Autodesk Inventor part; units mm, degrees
(part 2 of 3)
  spline S229 degree 2 poles (-22.9863, 76.6126) (-22.9863, 77.0351) (-22.389, 77.6357) (-21.9632, 77.6357) knots 0 0 0 1 2 2 2
  line L306 (-21.9632, 77.6357) -> (-21.1876, 77.6357)
  spline S230 degree 2 poles (-21.1876, 77.6357) (-20.9335, 77.6357) (-20.9335, 77.3882) knots 0 0 0 1 1 1
  spline S231 degree 2 poles (-20.9335, 77.3882) (-20.9335, 77.1374) (-21.1876, 77.1374) knots 0 0 0 1 1 1
  line L307 (-21.1876, 77.1374) -> (-21.9632, 77.1374)
  spline S232 degree 2 poles (-21.9632, 77.1374) (-22.1777, 77.1374) (-22.4847, 76.8304) (-22.4847, 76.6126) knots 0 0 0 1 2 2 2
  line L308 (-22.4847, 76.6126) -> (-22.4847, 74.672)
  spline S233 degree 2 poles (-22.4847, 74.672) (-22.4847, 74.4542) (-22.1777, 74.1473) (-21.9632, 74.1473) knots 0 0 0 1 2 2 2
  line L309 (-21.9632, 74.1473) -> (-21.1876, 74.1473)
  spline S234 degree 2 poles (-21.1876, 74.1473) (-20.9335, 74.1473) (-20.9335, 73.8997) knots 0 0 0 1 1 1
  spline S235 degree 2 poles (-20.9335, 73.8997) (-20.9335, 73.6489) (-21.1876, 73.6489) knots 0 0 0 1 1 1
  spline S236 degree 2 poles (-17.7355, 74.8667) (-17.7355, 74.3651) (-18.4517, 73.6489) (-18.9566, 73.6489) knots 0 0 0 1 2 2 2
  line L310 (-18.9566, 73.6489) -> (-20.1183, 73.6489)
  spline S237 degree 2 poles (-20.1183, 73.6489) (-20.2306, 73.6489) (-20.3692, 73.7875) (-20.3692, 73.8997) knots 0 0 0 1 2 2 2
  line L311 (-20.3692, 73.8997) -> (-20.3692, 77.3849)
  spline S238 degree 2 poles (-20.3692, 77.3849) (-20.3692, 77.4872) (-20.2207, 77.6357) (-20.1183, 77.6357) knots 0 0 0 1 2 2 2
  line L312 (-20.1183, 77.6357) -> (-18.9566, 77.6357)
  spline S239 degree 2 poles (-18.9566, 77.6357) (-18.5342, 77.6357) (-17.9302, 77.0318) (-17.9302, 76.6093) knots 0 0 0 1 2 2 2
  spline S240 degree 2 poles (-17.9302, 76.6093) (-17.9302, 76.1242) (-18.29, 75.8601) knots 0 0 0 1 1 1
  spline S241 degree 2 poles (-18.29, 75.8601) (-17.7355, 75.5433) (-17.7355, 74.8667) knots 0 0 0 1 1 1
  spline S242 degree 2 poles (-18.2372, 74.8667) (-18.2372, 75.1638) (-18.6596, 75.5862) (-18.9566, 75.5862) knots 0 0 0 1 2 2 2
  line L313 (-18.9566, 75.5862) -> (-19.8675, 75.5862)
  line L314 (-19.8675, 75.5862) -> (-19.8675, 74.1473)
  line L315 (-19.8675, 74.1473) -> (-18.9566, 74.1473)
  spline S243 degree 2 poles (-18.9566, 74.1473) (-18.6596, 74.1473) (-18.2372, 74.5697) (-18.2372, 74.8667) knots 0 0 0 1 2 2 2
  spline S244 degree 2 poles (-18.4319, 76.6126) (-18.4319, 76.8271) (-18.7421, 77.1374) (-18.9566, 77.1374) knots 0 0 0 1 2 2 2
  line L316 (-18.9566, 77.1374) -> (-19.8675, 77.1374)
  line L317 (-19.8675, 77.1374) -> (-19.8675, 76.0846)
  line L318 (-19.8675, 76.0846) -> (-18.9566, 76.0846)
  spline S245 degree 2 poles (-18.9566, 76.0846) (-18.7421, 76.0846) (-18.4319, 76.3948) (-18.4319, 76.6126) knots 0 0 0 1 2 2 2
  spline S246 degree 2 poles (-14.7289, 73.8997) (-14.7289, 73.6489) (-14.9797, 73.6489) knots 0 0 0 1 1 1
  spline S247 degree 2 poles (-14.9797, 73.6489) (-15.2306, 73.6489) (-15.2306, 73.8997) knots 0 0 0 1 1 1
  line L319 (-15.2306, 73.8997) -> (-15.2306, 75.2001)
  line L320 (-15.2306, 75.2001) -> (-15.8081, 75.2001)
  line L321 (-15.8081, 75.2001) -> (-16.7091, 73.7644)
  spline S248 degree 2 poles (-16.7091, 73.7644) (-16.7817, 73.6456) (-16.917, 73.6456) knots 0 0 0 1 1 1
  spline S249 degree 2 poles (-16.917, 73.6456) (-17.016, 73.6456) (-17.1744, 73.7941) (-17.1744, 73.8964) knots 0 0 0 1 2 2 2
  spline S250 degree 2 poles (-17.1744, 73.8964) (-17.1744, 73.9624) (-17.1348, 74.0285) knots 0 0 0 1 1 1
  line L322 (-17.1348, 74.0285) -> (-16.3428, 75.2463)
  spline S251 degree 2 poles (-16.3428, 75.2463) (-16.6794, 75.3123) (-17.1711, 75.9261) (-17.1711, 76.3222) knots 0 0 0 1 2 2 2
  line L323 (-17.1711, 76.3222) -> (-17.1711, 76.5136)
  spline S252 degree 2 poles (-17.1711, 76.5136) (-17.1711, 76.979) (-16.5144, 77.6357) (-16.049, 77.6357) knots 0 0 0 1 2 2 2
  line L324 (-16.049, 77.6357) -> (-14.983, 77.6357)
  spline S253 degree 2 poles (-14.983, 77.6357) (-14.8807, 77.6357) (-14.7289, 77.4839) (-14.7289, 77.3849) knots 0 0 0 1 2 2 2
  line L325 (-14.7289, 77.3849) -> (-14.7289, 73.8997)
  line L326 (-15.2306, 75.6984) -> (-15.2306, 77.1374)
  line L327 (-15.2306, 77.1374) -> (-16.049, 77.1374)
  spline S254 degree 2 poles (-16.049, 77.1374) (-16.3032, 77.1374) (-16.6695, 76.771) (-16.6695, 76.5136) knots 0 0 0 1 2 2 2
  line L328 (-16.6695, 76.5136) -> (-16.6695, 76.3222)
  spline S255 degree 2 poles (-16.6695, 76.3222) (-16.6695, 76.0648) (-16.3032, 75.6984) (-16.049, 75.6984) knots 0 0 0 1 2 2 2
  line L329 (-16.049, 75.6984) -> (-15.2306, 75.6984)
  spline S256 degree 2 poles (-12.016, 74.6753) (-12.016, 74.2496) (-12.6134, 73.6489) (-13.0424, 73.6489) knots 0 0 0 1 2 2 2
  line L330 (-13.0424, 73.6489) -> (-13.1381, 73.6489)
  spline S257 degree 2 poles (-13.1381, 73.6489) (-13.7355, 73.6489) (-14.0325, 74.1605) knots 0 0 0 1 1 1
  spline S258 degree 2 poles (-14.0325, 74.1605) (-14.0721, 74.2265) (-14.0721, 74.2892) knots 0 0 0 1 1 1
  spline S259 degree 2 poles (-14.0721, 74.2892) (-14.0721, 74.3915) (-13.9104, 74.54) (-13.8114, 74.54) knots 0 0 0 1 2 2 2
  spline S260 degree 2 poles (-13.8114, 74.54) (-13.6761, 74.54) (-13.6299, 74.4377) knots 0 0 0 1 1 1
  spline S261 degree 2 poles (-13.6299, 74.4377) (-13.4451, 74.1473) (-13.1381, 74.1473) knots 0 0 0 1 1 1
  line L331 (-13.1381, 74.1473) -> (-13.0424, 74.1473)
  spline S262 degree 2 poles (-13.0424, 74.1473) (-12.8246, 74.1473) (-12.5177, 74.4575) (-12.5177, 74.672) knots 0 0 0 1 2 2 2
  line L332 (-12.5177, 74.672) -> (-12.5177, 75.0615)
  spline S263 degree 2 poles (-12.5177, 75.0615) (-12.5177, 75.276) (-12.8279, 75.5862) (-13.0424, 75.5862) knots 0 0 0 1 2 2 2
  line L333 (-13.0424, 75.5862) -> (-13.4286, 75.5862)
  spline S264 degree 2 poles (-13.4286, 75.5862) (-13.6794, 75.5862) (-13.6794, 75.837) knots 0 0 0 1 1 1
  spline S265 degree 2 poles (-13.6794, 75.837) (-13.6794, 76.0846) (-13.4286, 76.0846) knots 0 0 0 1 1 1
  line L334 (-13.4286, 76.0846) -> (-12.8807, 76.0846)
  spline S266 degree 2 poles (-12.8807, 76.0846) (-12.7223, 76.1242) (-12.5177, 76.3915) (-12.5177, 76.5598) knots 0 0 0 1 2 2 2
  spline S267 degree 2 poles (-12.5177, 76.5598) (-12.5177, 76.8007) (-12.8576, 77.1374) (-13.0985, 77.1374) knots 0 0 0 1 2 2 2
  spline S268 degree 2 poles (-13.0985, 77.1374) (-13.3032, 77.1374) (-13.4649, 76.9988) knots 0 0 0 1 1 1
  spline S269 degree 2 poles (-13.4649, 76.9988) (-13.5408, 76.9393) (-13.6233, 76.9393) knots 0 0 0 1 1 1
  spline S270 degree 2 poles (-13.6233, 76.9393) (-13.7256, 76.9393) (-13.8774, 77.0978) (-13.8774, 77.1968) knots 0 0 0 1 2 2 2
  spline S271 degree 2 poles (-13.8774, 77.1968) (-13.8774, 77.3024) (-13.6893, 77.3948) knots 0 0 0 1 1 1
  spline S272 degree 2 poles (-13.6893, 77.3948) (-13.4814, 77.6357) (-13.0985, 77.6357) knots 0 0 0 1 1 1
  spline S273 degree 2 poles (-13.0985, 77.6357) (-12.6464, 77.6357) (-12.016, 77.0087) (-12.016, 76.5598) knots 0 0 0 1 2 2 2
  spline S274 degree 2 poles (-12.016, 76.5598) (-12.016, 76.0681) (-12.3791, 75.8172) knots 0 0 0 1 1 1
  spline S275 degree 2 poles (-12.3791, 75.8172) (-12.016, 75.5499) (-12.016, 75.0615) knots 0 0 0 1 1 1
  line L335 (-12.016, 75.0615) -> (-12.016, 74.6753)
  spline S276 degree 2 poles (-8.9104, 74.672) (-8.9104, 74.2463) (-9.5111, 73.6489) (-9.9401, 73.6489) knots 0 0 0 1 2 2 2
  line L336 (-9.9401, 73.6489) -> (-11.1018, 73.6489)
  spline S277 degree 2 poles (-11.1018, 73.6489) (-11.2041, 73.6489) (-11.3527, 73.7974) (-11.3527, 73.8997) knots 0 0 0 1 2 2 2
  line L337 (-11.3527, 73.8997) -> (-11.3527, 77.3849)
  spline S278 degree 2 poles (-11.3527, 77.3849) (-11.3527, 77.6357) (-11.1018, 77.6357) knots 0 0 0 1 1 1
  spline S279 degree 2 poles (-11.1018, 77.6357) (-10.851, 77.6357) (-10.851, 77.3849) knots 0 0 0 1 1 1
  line L338 (-10.851, 77.3849) -> (-10.851, 76.0846)
  line L339 (-10.851, 76.0846) -> (-9.9401, 76.0846)
  spline S280 degree 2 poles (-9.9401, 76.0846) (-9.5111, 76.0846) (-8.9104, 75.4839) (-8.9104, 75.0615) knots 0 0 0 1 2 2 2
  line L340 (-8.9104, 75.0615) -> (-8.9104, 74.672)
  line L341 (-9.4121, 74.672) -> (-9.4121, 75.0615)
  spline S281 degree 2 poles (-9.4121, 75.0615) (-9.4121, 75.276) (-9.7223, 75.5862) (-9.9401, 75.5862) knots 0 0 0 1 2 2 2
  line L342 (-9.9401, 75.5862) -> (-10.851, 75.5862)
  line L343 (-10.851, 75.5862) -> (-10.851, 74.1473)
  line L344 (-10.851, 74.1473) -> (-9.9401, 74.1473)
  spline S282 degree 2 poles (-9.9401, 74.1473) (-9.7223, 74.1473) (-9.4121, 74.4575) (-9.4121, 74.672) knots 0 0 0 1 2 2 2
  line L345 (-22.255, 49.6974) -> (-23.8504, 49.6974)
  spline S283 degree 2 poles (-23.8504, 49.6974) (-24.0502, 49.6974) (-24.0502, 49.8972) knots 0 0 0 1 1 1
  line L346 (-24.0502, 49.8972) -> (-24.0502, 53.4842)
  spline S284 degree 2 poles (-24.0502, 53.4842) (-24.0502, 53.6841) (-23.8504, 53.6841) knots 0 0 0 1 1 1
  spline S285 degree 2 poles (-23.8504, 53.6841) (-23.6506, 53.6841) (-23.6506, 53.4842) knots 0 0 0 1 1 1
  line L347 (-23.6506, 53.4842) -> (-23.6506, 50.0971)
  line L348 (-23.6506, 50.0971) -> (-22.255, 50.0971)
  spline S286 degree 2 poles (-22.255, 50.0971) (-22.0552, 50.0971) (-22.0552, 49.8972) knots 0 0 0 1 1 1
  spline S287 degree 2 poles (-22.0552, 49.8972) (-22.0552, 49.6974) (-22.255, 49.6974) knots 0 0 0 1 1 1
  spline S288 degree 2 poles (-18.8679, 50.6932) (-18.8679, 50.2802) (-19.4507, 49.6974) (-19.8637, 49.6974) knots 0 0 0 1 2 2 2
  line L349 (-19.8637, 49.6974) -> (-20.2634, 49.6974)
  spline S289 degree 2 poles (-20.2634, 49.6974) (-20.6764, 49.6974) (-21.2592, 50.2802) (-21.2592, 50.6932) knots 0 0 0 1 2 2 2
  line L350 (-21.2592, 50.6932) -> (-21.2592, 52.6882)
  spline S290 degree 2 poles (-21.2592, 52.6882) (-21.2592, 53.0979) (-20.6764, 53.6841) (-20.2634, 53.6841) knots 0 0 0 1 2 2 2
  line L351 (-20.2634, 53.6841) -> (-19.8637, 53.6841)
  spline S291 degree 2 poles (-19.8637, 53.6841) (-19.4507, 53.6841) (-18.8679, 53.0979) (-18.8679, 52.6882) knots 0 0 0 1 2 2 2
  line L352 (-18.8679, 52.6882) -> (-18.8679, 50.6932)
  line L353 (-19.2675, 50.6932) -> (-19.2675, 52.6882)
  spline S292 degree 2 poles (-19.2675, 52.6882) (-19.2675, 52.9347) (-19.6172, 53.2844) (-19.8637, 53.2844) knots 0 0 0 1 2 2 2
  line L354 (-19.8637, 53.2844) -> (-20.2634, 53.2844)
  spline S293 degree 2 poles (-20.2634, 53.2844) (-20.5098, 53.2844) (-20.8595, 52.9347) (-20.8595, 52.6882) knots 0 0 0 1 2 2 2
  line L355 (-20.8595, 52.6882) -> (-20.8595, 50.6932)
  spline S294 degree 2 poles (-20.8595, 50.6932) (-20.8595, 50.4468) (-20.5098, 50.0971) (-20.2634, 50.0971) knots 0 0 0 1 2 2 2
  line L356 (-20.2634, 50.0971) -> (-19.8637, 50.0971)
  spline S295 degree 2 poles (-19.8637, 50.0971) (-19.6172, 50.0971) (-19.2675, 50.4468) (-19.2675, 50.6932) knots 0 0 0 1 2 2 2
  spline S296 degree 2 poles (-15.6772, 52.4884) (-15.6772, 52.0821) (-16.1635, 51.4493) (-16.5431, 51.3394) knots 0 0 0 1 2 2 2
  line L357 (-16.5431, 51.3394) -> (-15.7105, 50.0005)
  spline S297 degree 2 poles (-15.7105, 50.0005) (-15.6739, 49.9439) (-15.6739, 49.8939) knots 0 0 0 1 1 1
  spline S298 degree 2 poles (-15.6739, 49.8939) (-15.6739, 49.814) (-15.8038, 49.6941) (-15.8837, 49.6941) knots 0 0 0 1 2 2 2
  spline S299 degree 2 poles (-15.8837, 49.6941) (-15.9836, 49.6941) (-16.0436, 49.7906) knots 0 0 0 1 1 1
  line L358 (-16.0436, 49.7906) -> (-16.9828, 51.2927)
  line L359 (-16.9828, 51.2927) -> (-17.6689, 51.2927)
  line L360 (-17.6689, 51.2927) -> (-17.6689, 49.8972)
  spline S300 degree 2 poles (-17.6689, 49.8972) (-17.6689, 49.6974) (-17.8687, 49.6974) knots 0 0 0 1 1 1
  spline S301 degree 2 poles (-17.8687, 49.6974) (-18.0685, 49.6974) (-18.0685, 49.8972) knots 0 0 0 1 1 1
  line L361 (-18.0685, 49.8972) -> (-18.0685, 53.4842)
  spline S302 degree 2 poles (-18.0685, 53.4842) (-18.0685, 53.5642) (-17.9486, 53.6841) (-17.8687, 53.6841) knots 0 0 0 1 2 2 2
  line L362 (-17.8687, 53.6841) -> (-16.8729, 53.6841)
  spline S303 degree 2 poles (-16.8729, 53.6841) (-16.3799, 53.6841) (-15.6772, 52.9813) (-15.6772, 52.4884) knots 0 0 0 1 2 2 2
  spline S304 degree 2 poles (-16.0769, 52.4884) (-16.0769, 52.8181) (-16.5431, 53.2844) (-16.8729, 53.2844) knots 0 0 0 1 2 2 2
  line L363 (-16.8729, 53.2844) -> (-17.6689, 53.2844)
  line L364 (-17.6689, 53.2844) -> (-17.6689, 51.6924)
  line L365 (-17.6689, 51.6924) -> (-16.8729, 51.6924)
  spline S305 degree 2 poles (-16.8729, 51.6924) (-16.5431, 51.6924) (-16.0769, 52.1587) (-16.0769, 52.4884) knots 0 0 0 1 2 2 2
  line L366 (-14.1818, 50.6999) -> (-14.4682, 49.8373)
  spline S306 degree 2 poles (-14.4682, 49.8373) (-14.5115, 49.7007) (-14.6481, 49.7007) knots 0 0 0 1 1 1
  spline S307 degree 2 poles (-14.6481, 49.7007) (-14.8546, 49.7007) (-14.8546, 49.8906) knots 0 0 0 1 1 1
  spline S308 degree 2 poles (-14.8546, 49.8906) (-14.8546, 49.9272) (-14.8412, 49.9638) knots 0 0 0 1 1 1
  line L367 (-14.8412, 49.9638) -> (-13.6422, 53.5542)
  spline S309 degree 2 poles (-13.6422, 53.5542) (-13.5856, 53.724) (-13.4557, 53.724) knots 0 0 0 1 1 1
  spline S310 degree 2 poles (-13.4557, 53.724) (-13.3225, 53.724) (-13.2692, 53.5542) knots 0 0 0 1 1 1
  line L368 (-13.2692, 53.5542) -> (-12.0702, 49.9638)
  spline S311 degree 2 poles (-12.0702, 49.9638) (-12.0602, 49.9272) (-12.0602, 49.8906) knots 0 0 0 1 1 1
  spline S312 degree 2 poles (-12.0602, 49.8906) (-12.0602, 49.7007) (-12.2667, 49.7007) knots 0 0 0 1 1 1
  spline S313 degree 2 poles (-12.2667, 49.7007) (-12.4033, 49.7007) (-12.4466, 49.8373) knots 0 0 0 1 1 1
  line L369 (-12.4466, 49.8373) -> (-12.733, 50.6999)
  line L370 (-12.733, 50.6999) -> (-14.1818, 50.6999)
  line L371 (-12.8695, 51.1062) -> (-13.4557, 52.8648)
  line L372 (-13.4557, 52.8648) -> (-14.0452, 51.1062)
  line L373 (-14.0452, 51.1062) -> (-12.8695, 51.1062)
  line L374 (16.4573, 53.5131) -> (15.6613, 49.9261)
  spline S314 degree 2 poles (15.6613, 49.9261) (15.6247, 49.7662) (15.4682, 49.7662) knots 0 0 0 1 1 1
  spline S315 degree 2 poles (15.4682, 49.7662) (15.325, 49.7662) (15.2783, 49.9027) knots 0 0 0 1 1 1
  line L375 (15.2783, 49.9027) -> (14.6688, 51.5813)
  line L376 (14.6688, 51.5813) -> (14.056, 49.9027)
  spline S316 degree 2 poles (14.056, 49.9027) (14.0094, 49.7662) (13.8695, 49.7662) knots 0 0 0 1 1 1
  spline S317 degree 2 poles (13.8695, 49.7662) (13.7096, 49.7662) (13.673, 49.9261) knots 0 0 0 1 1 1
  line L377 (13.673, 49.9261) -> (12.877, 53.5131)
  spline S318 degree 2 poles (12.877, 53.5131) (12.8737, 53.5364) (12.8737, 53.5664) knots 0 0 0 1 1 1
  spline S319 degree 2 poles (12.8737, 53.5664) (12.8737, 53.7562) (13.0768, 53.7562) knots 0 0 0 1 1 1
  spline S320 degree 2 poles (13.0768, 53.7562) (13.23, 53.7562) (13.2667, 53.5997) knots 0 0 0 1 1 1
  line L378 (13.2667, 53.5997) -> (13.9161, 50.6821)
  line L379 (13.9161, 50.6821) -> (14.479, 52.2308)
  spline S321 degree 2 poles (14.479, 52.2308) (14.5389, 52.394) (14.6688, 52.394) knots 0 0 0 1 1 1
  spline S322 degree 2 poles (14.6688, 52.394) (14.7954, 52.394) (14.8553, 52.2308) knots 0 0 0 1 1 1
  line L380 (14.8553, 52.2308) -> (15.4182, 50.6821)
  line L381 (15.4182, 50.6821) -> (16.0677, 53.5997)
  spline S323 degree 2 poles (16.0677, 53.5997) (16.1043, 53.7562) (16.2575, 53.7562) knots 0 0 0 1 1 1
  spline S324 degree 2 poles (16.2575, 53.7562) (16.4607, 53.7562) (16.4607, 53.5664) knots 0 0 0 1 1 1
  spline S325 degree 2 poles (16.4607, 53.5664) (16.4607, 53.5364) (16.4573, 53.5131) knots 0 0 0 1 1 1
  spline S326 degree 2 poles (17.6597, 49.9694) (17.6597, 49.7695) (17.4598, 49.7695) knots 0 0 0 1 1 1
  spline S327 degree 2 poles (17.4598, 49.7695) (17.26, 49.7695) (17.26, 49.9694) knots 0 0 0 1 1 1
  line L382 (17.26, 49.9694) -> (17.26, 53.5564)
  spline S328 degree 2 poles (17.26, 53.5564) (17.26, 53.7562) (17.4598, 53.7562) knots 0 0 0 1 1 1
  spline S329 degree 2 poles (17.4598, 53.7562) (17.6597, 53.7562) (17.6597, 53.5564) knots 0 0 0 1 1 1
  line L383 (17.6597, 53.5564) -> (17.6597, 49.9694)
  spline S330 degree 2 poles (20.847, 52.5605) (20.847, 52.1542) (20.3608, 51.5214) (19.9811, 51.4115) knots 0 0 0 1 2 2 2
  line L384 (19.9811, 51.4115) -> (20.8137, 50.0726)
  spline S331 degree 2 poles (20.8137, 50.0726) (20.8503, 50.016) (20.8503, 49.966) knots 0 0 0 1 1 1
  spline S332 degree 2 poles (20.8503, 49.966) (20.8503, 49.8861) (20.7205, 49.7662) (20.6405, 49.7662) knots 0 0 0 1 2 2 2
  spline S333 degree 2 poles (20.6405, 49.7662) (20.5406, 49.7662) (20.4807, 49.8628) knots 0 0 0 1 1 1
  line L385 (20.4807, 49.8628) -> (19.5414, 51.3649)
  line L386 (19.5414, 51.3649) -> (18.8553, 51.3649)
  line L387 (18.8553, 51.3649) -> (18.8553, 49.9694)
  spline S334 degree 2 poles (18.8553, 49.9694) (18.8553, 49.7695) (18.6555, 49.7695) knots 0 0 0 1 1 1
  spline S335 degree 2 poles (18.6555, 49.7695) (18.4557, 49.7695) (18.4557, 49.9694) knots 0 0 0 1 1 1
  line L388 (18.4557, 49.9694) -> (18.4557, 53.5564)
  spline S336 degree 2 poles (18.4557, 53.5564) (18.4557, 53.6363) (18.5756, 53.7562) (18.6555, 53.7562) knots 0 0 0 1 2 2 2
  line L389 (18.6555, 53.7562) -> (19.6513, 53.7562)
  spline S337 degree 2 poles (19.6513, 53.7562) (20.1443, 53.7562) (20.847, 53.0535) (20.847, 52.5605) knots 0 0 0 1 2 2 2
  spline S338 degree 2 poles (20.4474, 52.5605) (20.4474, 52.8903) (19.9811, 53.3565) (19.6513, 53.3565) knots 0 0 0 1 2 2 2
  line L390 (19.6513, 53.3565) -> (18.8553, 53.3565)
  line L391 (18.8553, 53.3565) -> (18.8553, 51.7645)
  line L392 (18.8553, 51.7645) -> (19.6513, 51.7645)
  spline S339 degree 2 poles (19.6513, 51.7645) (19.9811, 51.7645) (20.4474, 52.2308) (20.4474, 52.5605) knots 0 0 0 1 2 2 2
  line L393 (22.046, 52.1609) -> (23.0485, 52.1609)
  spline S340 degree 2 poles (23.0485, 52.1609) (23.245, 52.1609) (23.245, 51.961) knots 0 0 0 1 1 1
  spline S341 degree 2 poles (23.245, 51.961) (23.245, 51.7612) (23.0485, 51.7612) knots 0 0 0 1 1 1
  line L394 (23.0485, 51.7612) -> (22.046, 51.7612)
  line L395 (22.046, 51.7612) -> (22.046, 50.1692)
  line L396 (22.046, 50.1692) -> (23.4449, 50.1692)
  spline S342 degree 2 poles (23.4449, 50.1692) (23.6447, 50.1692) (23.6447, 49.9694) knots 0 0 0 1 1 1
  spline S343 degree 2 poles (23.6447, 49.9694) (23.6447, 49.7695) (23.4449, 49.7695) knots 0 0 0 1 1 1
  line L397 (23.4449, 49.7695) -> (21.8462, 49.7695)
  spline S344 degree 2 poles (21.8462, 49.7695) (21.6464, 49.7695) (21.6464, 49.956) knots 0 0 0 1 1 1
  line L398 (21.6464, 49.956) -> (21.6464, 53.5564)
  spline S345 degree 2 poles (21.6464, 53.5564) (21.6464, 53.7562) (21.8462, 53.7562) knots 0 0 0 1 1 1
  line L399 (21.8462, 53.7562) -> (23.4449, 53.7562)
  spline S346 degree 2 poles (23.4449, 53.7562) (23.6447, 53.7562) (23.6447, 53.5564) knots 0 0 0 1 1 1
  spline S347 degree 2 poles (23.6447, 53.5564) (23.6447, 53.3565) (23.4449, 53.3565) knots 0 0 0 1 1 1
  line L400 (23.4449, 53.3565) -> (22.046, 53.3565)
  line L401 (22.046, 53.3565) -> (22.046, 52.1609)
  line L402 (-22.2779, 42.1598) -> (-23.2729, 37.676)
  spline S348 degree 2 poles (-23.2729, 37.676) (-23.3187, 37.4762) (-23.5144, 37.4762) knots 0 0 0 1 1 1
  spline S349 degree 2 poles (-23.5144, 37.4762) (-23.6934, 37.4762) (-23.7517, 37.6469) knots 0 0 0 1 1 1
  line L403 (-23.7517, 37.6469) -> (-24.5136, 39.7451)
  line L404 (-24.5136, 39.7451) -> (-25.2796, 37.6469)
  spline S350 degree 2 poles (-25.2796, 37.6469) (-25.3379, 37.4762) (-25.5127, 37.4762) knots 0 0 0 1 1 1
  spline S351 degree 2 poles (-25.5127, 37.4762) (-25.7126, 37.4762) (-25.7584, 37.676) knots 0 0 0 1 1 1
  line L405 (-25.7584, 37.676) -> (-26.7534, 42.1598)
  spline S352 degree 2 poles (-26.7534, 42.1598) (-26.7575, 42.1889) (-26.7575, 42.2264) knots 0 0 0 1 1 1
  spline S353 degree 2 poles (-26.7575, 42.2264) (-26.7575, 42.4637) (-26.5036, 42.4637) knots 0 0 0 1 1 1
  spline S354 degree 2 poles (-26.5036, 42.4637) (-26.3121, 42.4637) (-26.2663, 42.268) knots 0 0 0 1 1 1
  line L406 (-26.2663, 42.268) -> (-25.4545, 38.6211)
  line L407 (-25.4545, 38.6211) -> (-24.7509, 40.557)
  spline S355 degree 2 poles (-24.7509, 40.557) (-24.6759, 40.761) (-24.5136, 40.761) knots 0 0 0 1 1 1
  spline S356 degree 2 poles (-24.5136, 40.761) (-24.3554, 40.761) (-24.2804, 40.557) knots 0 0 0 1 1 1
  line L408 (-24.2804, 40.557) -> (-23.5769, 38.6211)
  line L409 (-23.5769, 38.6211) -> (-22.765, 42.268)
  spline S357 degree 2 poles (-22.765, 42.268) (-22.7192, 42.4637) (-22.5277, 42.4637) knots 0 0 0 1 1 1
  spline S358 degree 2 poles (-22.5277, 42.4637) (-22.2738, 42.4637) (-22.2738, 42.2264) knots 0 0 0 1 1 1
  spline S359 degree 2 poles (-22.2738, 42.2264) (-22.2738, 42.1889) (-22.2779, 42.1598) knots 0 0 0 1 1 1
  spline S360 degree 2 poles (-20.775, 37.7301) (-20.775, 37.4804) (-21.0248, 37.4804) knots 0 0 0 1 1 1
  spline S361 degree 2 poles (-21.0248, 37.4804) (-21.2746, 37.4804) (-21.2746, 37.7301) knots 0 0 0 1 1 1
  line L410 (-21.2746, 37.7301) -> (-21.2746, 42.2139)
  spline S362 degree 2 poles (-21.2746, 42.2139) (-21.2746, 42.4637) (-21.0248, 42.4637) knots 0 0 0 1 1 1
  spline S363 degree 2 poles (-21.0248, 42.4637) (-20.775, 42.4637) (-20.775, 42.2139) knots 0 0 0 1 1 1
  line L411 (-20.775, 42.2139) -> (-20.775, 37.7301)
  spline S364 degree 2 poles (-16.7909, 40.9691) (-16.7909, 40.4612) (-17.3987, 39.6702) (-17.8733, 39.5328) knots 0 0 0 1 2 2 2
  line L412 (-17.8733, 39.5328) -> (-16.8325, 37.8592)
  spline S365 degree 2 poles (-16.8325, 37.8592) (-16.7867, 37.7884) (-16.7867, 37.726) knots 0 0 0 1 1 1
  spline S366 degree 2 poles (-16.7867, 37.726) (-16.7867, 37.6261) (-16.9491, 37.4762) (-17.049, 37.4762) knots 0 0 0 1 2 2 2
  spline S367 degree 2 poles (-17.049, 37.4762) (-17.1739, 37.4762) (-17.2488, 37.5969) knots 0 0 0 1 1 1
  line L413 (-17.2488, 37.5969) -> (-18.4228, 39.4745)
  line L414 (-18.4228, 39.4745) -> (-19.2804, 39.4745)
  line L415 (-19.2804, 39.4745) -> (-19.2804, 37.7301)
  spline S368 degree 2 poles (-19.2804, 37.7301) (-19.2804, 37.4804) (-19.5302, 37.4804) knots 0 0 0 1 1 1
  spline S369 degree 2 poles (-19.5302, 37.4804) (-19.78, 37.4804) (-19.78, 37.7301) knots 0 0 0 1 1 1
  line L416 (-19.78, 37.7301) -> (-19.78, 42.2139)
  spline S370 degree 2 poles (-19.78, 42.2139) (-19.78, 42.3138) (-19.6302, 42.4637) (-19.5302, 42.4637) knots 0 0 0 1 2 2 2
  line L417 (-19.5302, 42.4637) -> (-18.2854, 42.4637)
  spline S371 degree 2 poles (-18.2854, 42.4637) (-17.6693, 42.4637) (-16.7909, 41.5853) (-16.7909, 40.9691) knots 0 0 0 1 2 2 2
  spline S372 degree 2 poles (-17.2904, 40.9691) (-17.2904, 41.3813) (-17.8733, 41.9641) (-18.2854, 41.9641) knots 0 0 0 1 2 2 2
  line L418 (-18.2854, 41.9641) -> (-19.2804, 41.9641)
  line L419 (-19.2804, 41.9641) -> (-19.2804, 39.9741)
  line L420 (-19.2804, 39.9741) -> (-18.2854, 39.9741)
  spline S373 degree 2 poles (-18.2854, 39.9741) (-17.8733, 39.9741) (-17.2904, 40.557) (-17.2904, 40.9691) knots 0 0 0 1 2 2 2
  line L421 (-15.2921, 40.4695) -> (-14.039, 40.4695)
  spline S374 degree 2 poles (-14.039, 40.4695) (-13.7933, 40.4695) (-13.7933, 40.2197) knots 0 0 0 1 1 1
  spline S375 degree 2 poles (-13.7933, 40.2197) (-13.7933, 39.97) (-14.039, 39.97) knots 0 0 0 1 1 1
  line L422 (-14.039, 39.97) -> (-15.2921, 39.97)
  line L423 (-15.2921, 39.97) -> (-15.2921, 37.9799)
  line L424 (-15.2921, 37.9799) -> (-13.5436, 37.9799)
  spline S376 degree 2 poles (-13.5436, 37.9799) (-13.2938, 37.9799) (-13.2938, 37.7301) knots 0 0 0 1 1 1
  spline S377 degree 2 poles (-13.2938, 37.7301) (-13.2938, 37.4804) (-13.5436, 37.4804) knots 0 0 0 1 1 1
  line L425 (-13.5436, 37.4804) -> (-15.5419, 37.4804)
  spline S378 degree 2 poles (-15.5419, 37.4804) (-15.7917, 37.4804) (-15.7917, 37.7135) knots 0 0 0 1 1 1
  line L426 (-15.7917, 37.7135) -> (-15.7917, 42.2139)
  spline S379 degree 2 poles (-15.7917, 42.2139) (-15.7917, 42.4637) (-15.5419, 42.4637) knots 0 0 0 1 1 1
  line L427 (-15.5419, 42.4637) -> (-13.5436, 42.4637)
  spline S380 degree 2 poles (-13.5436, 42.4637) (-13.2938, 42.4637) (-13.2938, 42.2139) knots 0 0 0 1 1 1
  spline S381 degree 2 poles (-13.2938, 42.2139) (-13.2938, 41.9641) (-13.5436, 41.9641) knots 0 0 0 1 1 1
  line L428 (-13.5436, 41.9641) -> (-15.2921, 41.9641)
  line L429 (-15.2921, 41.9641) -> (-15.2921, 40.4695)
  line L430 (-7.0698, 37.4804) -> (-8.0648, 37.4804)
  spline S382 degree 2 poles (-8.0648, 37.4804) (-8.5852, 37.4804) (-9.3137, 38.2089) (-9.3137, 38.7252) knots 0 0 0 1 2 2 2
  line L431 (-9.3137, 38.7252) -> (-9.3137, 41.2189)
  spline S383 degree 2 poles (-9.3137, 41.2189) (-9.3137, 41.7351) (-8.5852, 42.4637) (-8.0648, 42.4637) knots 0 0 0 1 2 2 2
  line L432 (-8.0648, 42.4637) -> (-7.0698, 42.4637)
  spline S384 degree 2 poles (-7.0698, 42.4637) (-6.82, 42.4637) (-6.82, 42.2139) knots 0 0 0 1 1 1
  spline S385 degree 2 poles (-6.82, 42.2139) (-6.82, 41.9641) (-7.0698, 41.9641) knots 0 0 0 1 1 1
  line L433 (-7.0698, 41.9641) -> (-8.0648, 41.9641)
  spline S386 degree 2 poles (-8.0648, 41.9641) (-8.377, 41.9641) (-8.8142, 41.527) (-8.8142, 41.2189) knots 0 0 0 1 2 2 2
  line L434 (-8.8142, 41.2189) -> (-8.8142, 38.7252)
  spline S387 degree 2 poles (-8.8142, 38.7252) (-8.8142, 38.4171) (-8.377, 37.9799) (-8.0648, 37.9799) knots 0 0 0 1 2 2 2
  line L435 (-8.0648, 37.9799) -> (-7.0698, 37.9799)
  spline S388 degree 2 poles (-7.0698, 37.9799) (-6.82, 37.9799) (-6.82, 37.7301) knots 0 0 0 1 1 1
  spline S389 degree 2 poles (-6.82, 37.7301) (-6.82, 37.4804) (-7.0698, 37.4804) knots 0 0 0 1 1 1
  spline S390 degree 2 poles (-2.8358, 38.7252) (-2.8358, 38.2089) (-3.5644, 37.4804) (-4.0806, 37.4804) knots 0 0 0 1 2 2 2
  line L436 (-4.0806, 37.4804) -> (-4.5802, 37.4804)
  spline S391 degree 2 poles (-4.5802, 37.4804) (-5.0964, 37.4804) (-5.825, 38.2089) (-5.825, 38.7252) knots 0 0 0 1 2 2 2
  line L437 (-5.825, 38.7252) -> (-5.825, 41.2189)
  spline S392 degree 2 poles (-5.825, 41.2189) (-5.825, 41.731) (-5.0964, 42.4637) (-4.5802, 42.4637) knots 0 0 0 1 2 2 2
  line L438 (-4.5802, 42.4637) -> (-4.0806, 42.4637)
  spline S393 degree 2 poles (-4.0806, 42.4637) (-3.5644, 42.4637) (-2.8358, 41.731) (-2.8358, 41.2189) knots 0 0 0 1 2 2 2
  line L439 (-2.8358, 41.2189) -> (-2.8358, 38.7252)
  line L440 (-3.3354, 38.7252) -> (-3.3354, 41.2189)
  spline S394 degree 2 poles (-3.3354, 41.2189) (-3.3354, 41.527) (-3.7725, 41.9641) (-4.0806, 41.9641) knots 0 0 0 1 2 2 2
  line L441 (-4.0806, 41.9641) -> (-4.5802, 41.9641)
  spline S395 degree 2 poles (-4.5802, 41.9641) (-4.8883, 41.9641) (-5.3254, 41.527) (-5.3254, 41.2189) knots 0 0 0 1 2 2 2
  line L442 (-5.3254, 41.2189) -> (-5.3254, 38.7252)
  spline S396 degree 2 poles (-5.3254, 38.7252) (-5.3254, 38.4171) (-4.8883, 37.9799) (-4.5802, 37.9799) knots 0 0 0 1 2 2 2
  line L443 (-4.5802, 37.9799) -> (-4.0806, 37.9799)
  spline S397 degree 2 poles (-4.0806, 37.9799) (-3.7725, 37.9799) (-3.3354, 38.4171) (-3.3354, 38.7252) knots 0 0 0 1 2 2 2
  spline S398 degree 2 poles (1.1484, 37.7551) (1.1484, 37.4762) (0.9194, 37.4762) knots 0 0 0 1 1 1
  spline S399 degree 2 poles (0.9194, 37.4762) (0.7695, 37.4762) (0.6779, 37.6344) knots 0 0 0 1 1 1
  line L444 (0.6779, 37.6344) -> (-1.3371, 41.2231)
  line L445 (-1.3371, 41.2231) -> (-1.3371, 37.7301)
  spline S400 degree 2 poles (-1.3371, 37.7301) (-1.3371, 37.4804) (-1.5869, 37.4804) knots 0 0 0 1 1 1
  spline S401 degree 2 poles (-1.5869, 37.4804) (-1.8366, 37.4804) (-1.8366, 37.7301) knots 0 0 0 1 1 1
  line L446 (-1.8366, 37.7301) -> (-1.8366, 42.1889)
  spline S402 degree 2 poles (-1.8366, 42.1889) (-1.8366, 42.4637) (-1.5993, 42.4637) knots 0 0 0 1 1 1
  spline S403 degree 2 poles (-1.5993, 42.4637) (-1.4495, 42.4637) (-1.3662, 42.3097) knots 0 0 0 1 1 1
  line L447 (-1.3662, 42.3097) -> (0.6488, 38.721)
  line L448 (0.6488, 38.721) -> (0.6488, 42.2139)
  spline S404 degree 2 poles (0.6488, 42.2139) (0.6488, 42.4637) (0.8986, 42.4637) knots 0 0 0 1 1 1
  spline S405 degree 2 poles (0.8986, 42.4637) (1.1484, 42.4637) (1.1484, 42.2139) knots 0 0 0 1 1 1
  line L449 (1.1484, 42.2139) -> (1.1484, 37.7551)
  spline S406 degree 2 poles (5.1367, 37.7551) (5.1367, 37.4762) (4.9077, 37.4762) knots 0 0 0 1 1 1
  spline S407 degree 2 poles (4.9077, 37.4762) (4.7579, 37.4762) (4.6663, 37.6344) knots 0 0 0 1 1 1
  line L450 (4.6663, 37.6344) -> (2.6513, 41.2231)
  line L451 (2.6513, 41.2231) -> (2.6513, 37.7301)
  spline S408 degree 2 poles (2.6513, 37.7301) (2.6513, 37.4804) (2.4015, 37.4804) knots 0 0 0 1 1 1
  spline S409 degree 2 poles (2.4015, 37.4804) (2.1517, 37.4804) (2.1517, 37.7301) knots 0 0 0 1 1 1
  line L452 (2.1517, 37.7301) -> (2.1517, 42.1889)
  spline S410 degree 2 poles (2.1517, 42.1889) (2.1517, 42.4637) (2.389, 42.4637) knots 0 0 0 1 1 1
  spline S411 degree 2 poles (2.389, 42.4637) (2.5389, 42.4637) (2.6221, 42.3097) knots 0 0 0 1 1 1
  line L453 (2.6221, 42.3097) -> (4.6371, 38.721)
  line L454 (4.6371, 38.721) -> (4.6371, 42.2139)
  spline S412 degree 2 poles (4.6371, 42.2139) (4.6371, 42.4637) (4.8869, 42.4637) knots 0 0 0 1 1 1
  spline S413 degree 2 poles (4.8869, 42.4637) (5.1367, 42.4637) (5.1367, 42.2139) knots 0 0 0 1 1 1
  line L455 (5.1367, 42.2139) -> (5.1367, 37.7551)
  line L456 (6.6396, 40.4695) -> (7.8927, 40.4695)
  spline S414 degree 2 poles (7.8927, 40.4695) (8.1384, 40.4695) (8.1384, 40.2197) knots 0 0 0 1 1 1
  spline S415 degree 2 poles (8.1384, 40.2197) (8.1384, 39.97) (7.8927, 39.97) knots 0 0 0 1 1 1
  line L457 (7.8927, 39.97) -> (6.6396, 39.97)
  line L458 (6.6396, 39.97) -> (6.6396, 37.9799)
  line L459 (6.6396, 37.9799) -> (8.3882, 37.9799)
  spline S416 degree 2 poles (8.3882, 37.9799) (8.638, 37.9799) (8.638, 37.7301) knots 0 0 0 1 1 1
  spline S417 degree 2 poles (8.638, 37.7301) (8.638, 37.4804) (8.3882, 37.4804) knots 0 0 0 1 1 1
  line L460 (8.3882, 37.4804) -> (6.3898, 37.4804)
  spline S418 degree 2 poles (6.3898, 37.4804) (6.14, 37.4804) (6.14, 37.7135) knots 0 0 0 1 1 1
  line L461 (6.14, 37.7135) -> (6.14, 42.2139)
  spline S419 degree 2 poles (6.14, 42.2139) (6.14, 42.4637) (6.3898, 42.4637) knots 0 0 0 1 1 1
  line L462 (6.3898, 42.4637) -> (8.3882, 42.4637)
  spline S420 degree 2 poles (8.3882, 42.4637) (8.638, 42.4637) (8.638, 42.2139) knots 0 0 0 1 1 1
  spline S421 degree 2 poles (8.638, 42.2139) (8.638, 41.9641) (8.3882, 41.9641) knots 0 0 0 1 1 1
  line L463 (8.3882, 41.9641) -> (6.6396, 41.9641)
  line L464 (6.6396, 41.9641) -> (6.6396, 40.4695)
  line L465 (11.8728, 37.4804) -> (10.8778, 37.4804)
  spline S422 degree 2 poles (10.8778, 37.4804) (10.3574, 37.4804) (9.6288, 38.2089) (9.6288, 38.7252) knots 0 0 0 1 2 2 2
  line L466 (9.6288, 38.7252) -> (9.6288, 41.2189)
  spline S423 degree 2 poles (9.6288, 41.2189) (9.6288, 41.7351) (10.3574, 42.4637) (10.8778, 42.4637) knots 0 0 0 1 2 2 2
  line L467 (10.8778, 42.4637) -> (11.8728, 42.4637)
  spline S424 degree 2 poles (11.8728, 42.4637) (12.1226, 42.4637) (12.1226, 42.2139) knots 0 0 0 1 1 1
  spline S425 degree 2 poles (12.1226, 42.2139) (12.1226, 41.9641) (11.8728, 41.9641) knots 0 0 0 1 1 1
  line L468 (11.8728, 41.9641) -> (10.8778, 41.9641)
  spline S426 degree 2 poles (10.8778, 41.9641) (10.5655, 41.9641) (10.1284, 41.527) (10.1284, 41.2189) knots 0 0 0 1 2 2 2
  line L469 (10.1284, 41.2189) -> (10.1284, 38.7252)
  spline S427 degree 2 poles (10.1284, 38.7252) (10.1284, 38.4171) (10.5655, 37.9799) (10.8778, 37.9799) knots 0 0 0 1 2 2 2
  line L470 (10.8778, 37.9799) -> (11.8728, 37.9799)
  spline S428 degree 2 poles (11.8728, 37.9799) (12.1226, 37.9799) (12.1226, 37.7301) knots 0 0 0 1 1 1
  spline S429 degree 2 poles (12.1226, 37.7301) (12.1226, 37.4804) (11.8728, 37.4804) knots 0 0 0 1 1 1
  line L471 (14.3665, 41.9641) -> (13.3674, 41.9641)
  spline S430 degree 2 poles (13.3674, 41.9641) (13.1176, 41.9641) (13.1176, 42.2139) knots 0 0 0 1 1 1
  spline S431 degree 2 poles (13.1176, 42.2139) (13.1176, 42.4637) (13.3674, 42.4637) knots 0 0 0 1 1 1
  line L472 (13.3674, 42.4637) -> (15.8611, 42.4637)
  spline S432 degree 2 poles (15.8611, 42.4637) (16.1109, 42.4637) (16.1109, 42.2139) knots 0 0 0 1 1 1
  spline S433 degree 2 poles (16.1109, 42.2139) (16.1109, 41.9641) (15.8611, 41.9641) knots 0 0 0 1 1 1
  line L473 (15.8611, 41.9641) -> (14.8619, 41.9641)
  line L474 (14.8619, 41.9641) -> (14.8619, 37.7301)
  spline S434 degree 2 poles (14.8619, 37.7301) (14.8619, 37.4804) (14.6163, 37.4804) knots 0 0 0 1 1 1
  spline S435 degree 2 poles (14.6163, 37.4804) (14.3665, 37.4804) (14.3665, 37.7301) knots 0 0 0 1 1 1
  line L475 (14.3665, 37.7301) -> (14.3665, 41.9641)
  spline S436 degree 2 poles (17.6096, 37.7301) (17.6096, 37.4804) (17.3599, 37.4804) knots 0 0 0 1 1 1
  spline S437 degree 2 poles (17.3599, 37.4804) (17.1101, 37.4804) (17.1101, 37.7301) knots 0 0 0 1 1 1
  line L476 (17.1101, 37.7301) -> (17.1101, 42.2139)
  spline S438 degree 2 poles (17.1101, 42.2139) (17.1101, 42.4637) (17.3599, 42.4637) knots 0 0 0 1 1 1
  spline S439 degree 2 poles (17.3599, 42.4637) (17.6096, 42.4637) (17.6096, 42.2139) knots 0 0 0 1 1 1
  line L477 (17.6096, 42.2139) -> (17.6096, 37.7301)
  spline S440 degree 2 poles (21.5938, 38.7252) (21.5938, 38.2089) (20.8653, 37.4804) (20.349, 37.4804) knots 0 0 0 1 2 2 2
  line L478 (20.349, 37.4804) -> (19.8494, 37.4804)
  spline S441 degree 2 poles (19.8494, 37.4804) (19.3332, 37.4804) (18.6047, 38.2089) (18.6047, 38.7252) knots 0 0 0 1 2 2 2
  line L479 (18.6047, 38.7252) -> (18.6047, 41.2189)
  spline S442 degree 2 poles (18.6047, 41.2189) (18.6047, 41.731) (19.3332, 42.4637) (19.8494, 42.4637) knots 0 0 0 1 2 2 2
  line L480 (19.8494, 42.4637) -> (20.349, 42.4637)
  spline S443 degree 2 poles (20.349, 42.4637) (20.8653, 42.4637) (21.5938, 41.731) (21.5938, 41.2189) knots 0 0 0 1 2 2 2
  line L481 (21.5938, 41.2189) -> (21.5938, 38.7252)
  line L482 (21.0942, 38.7252) -> (21.0942, 41.2189)
  spline S444 degree 2 poles (21.0942, 41.2189) (21.0942, 41.527) (20.6571, 41.9641) (20.349, 41.9641) knots 0 0 0 1 2 2 2
  line L483 (20.349, 41.9641) -> (19.8494, 41.9641)
  spline S445 degree 2 poles (19.8494, 41.9641) (19.5414, 41.9641) (19.1042, 41.527) (19.1042, 41.2189) knots 0 0 0 1 2 2 2
  line L484 (19.1042, 41.2189) -> (19.1042, 38.7252)
  spline S446 degree 2 poles (19.1042, 38.7252) (19.1042, 38.4171) (19.5414, 37.9799) (19.8494, 37.9799) knots 0 0 0 1 2 2 2
  line L485 (19.8494, 37.9799) -> (20.349, 37.9799)
  spline S447 degree 2 poles (20.349, 37.9799) (20.6571, 37.9799) (21.0942, 38.4171) (21.0942, 38.7252) knots 0 0 0 1 2 2 2
  spline S448 degree 2 poles (25.578, 37.7551) (25.578, 37.4762) (25.349, 37.4762) knots 0 0 0 1 1 1
  spline S449 degree 2 poles (25.349, 37.4762) (25.1992, 37.4762) (25.1076, 37.6344) knots 0 0 0 1 1 1
  line L486 (25.1076, 37.6344) -> (23.0926, 41.2231)
  line L487 (23.0926, 41.2231) -> (23.0926, 37.7301)
  spline S450 degree 2 poles (23.0926, 37.7301) (23.0926, 37.4804) (22.8428, 37.4804) knots 0 0 0 1 1 1
  spline S451 degree 2 poles (22.8428, 37.4804) (22.593, 37.4804) (22.593, 37.7301) knots 0 0 0 1 1 1
  line L488 (22.593, 37.7301) -> (22.593, 42.1889)
  spline S452 degree 2 poles (22.593, 42.1889) (22.593, 42.4637) (22.8303, 42.4637) knots 0 0 0 1 1 1
  spline S453 degree 2 poles (22.8303, 42.4637) (22.9802, 42.4637) (23.0634, 42.3097) knots 0 0 0 1 1 1
  line L489 (23.0634, 42.3097) -> (25.0784, 38.721)
  line L490 (25.0784, 38.721) -> (25.0784, 42.2139)
  spline S454 degree 2 poles (25.0784, 42.2139) (25.0784, 42.4637) (25.3282, 42.4637) knots 0 0 0 1 1 1
  spline S455 degree 2 poles (25.3282, 42.4637) (25.578, 42.4637) (25.578, 42.2139) knots 0 0 0 1 1 1
  line L491 (25.578, 42.2139) -> (25.578, 37.7551)
  spline S456 degree 2 poles (-20.9359, 12.9488) (-20.9359, 12.698) (-21.1868, 12.698) knots 0 0 0 1 1 1
  spline S457 degree 2 poles (-21.1868, 12.698) (-21.4376, 12.698) (-21.4376, 12.9488) knots 0 0 0 1 1 1
  line L492 (-21.4376, 12.9488) -> (-21.4376, 14.6947)
  spline S458 degree 2 poles (-21.4376, 14.6947) (-21.4376, 14.8267) (-21.6356, 15.0247) (-21.7709, 15.0247) knots 0 0 0 1 2 2 2
  line L493 (-21.7709, 15.0247) -> (-22.4904, 15.0247)
  line L494 (-22.4904, 15.0247) -> (-22.4904, 12.9488)
  spline S459 degree 2 poles (-22.4904, 12.9488) (-22.4904, 12.698) (-22.7412, 12.698) knots 0 0 0 1 1 1
  spline S460 degree 2 poles (-22.7412, 12.698) (-22.992, 12.698) (-22.992, 12.9488) knots 0 0 0 1 1 1
  line L495 (-22.992, 12.9488) -> (-22.992, 15.2723)
  spline S461 degree 2 poles (-22.992, 15.2723) (-22.992, 15.5231) (-22.7412, 15.5231) knots 0 0 0 1 1 1
  line L496 (-22.7412, 15.5231) -> (-21.7709, 15.5231)
  spline S462 degree 2 poles (-21.7709, 15.5231) (-21.4244, 15.5231) (-20.9359, 15.0346) (-20.9359, 14.6914) knots 0 0 0 1 2 2 2
  line L497 (-20.9359, 14.6914) -> (-20.9359, 12.9488)
  line L498 (-18.7214, 12.698) -> (-19.4409, 12.698)
  spline S463 degree 2 poles (-19.4409, 12.698) (-19.7841, 12.698) (-20.2759, 13.1831) (-20.2759, 13.5297) knots 0 0 0 1 2 2 2
  line L499 (-20.2759, 13.5297) -> (-20.2759, 15.2723)
  spline S464 degree 2 poles (-20.2759, 15.2723) (-20.2759, 15.5231) (-20.025, 15.5231) knots 0 0 0 1 1 1
  spline S465 degree 2 poles (-20.025, 15.5231) (-19.7742, 15.5231) (-19.7742, 15.2723) knots 0 0 0 1 1 1
  line L500 (-19.7742, 15.2723) -> (-19.7742, 13.5297)
  spline S466 degree 2 poles (-19.7742, 13.5297) (-19.7742, 13.3911) (-19.5795, 13.1963) (-19.4442, 13.1963) knots 0 0 0 1 2 2 2
  line L501 (-19.4442, 13.1963) -> (-18.7214, 13.1963)
  line L502 (-18.7214, 13.1963) -> (-18.7214, 15.2723)
  spline S467 degree 2 poles (-18.7214, 15.2723) (-18.7214, 15.5231) (-18.4706, 15.5231) knots 0 0 0 1 1 1
  spline S468 degree 2 poles (-18.4706, 15.5231) (-18.2198, 15.5231) (-18.2198, 15.2723) knots 0 0 0 1 1 1
  line L503 (-18.2198, 15.2723) -> (-18.2198, 12.368)
  spline S469 degree 2 poles (-18.2198, 12.368) (-18.2198, 12.0214) (-18.7082, 11.5363) (-19.0547, 11.5363) knots 0 0 0 1 2 2 2
  line L504 (-19.0547, 11.5363) -> (-19.8336, 11.5363)
  spline S470 degree 2 poles (-19.8336, 11.5363) (-20.0845, 11.5363) (-20.0845, 11.7871) knots 0 0 0 1 1 1
  spline S471 degree 2 poles (-20.0845, 11.7871) (-20.0845, 12.0346) (-19.8336, 12.0346) knots 0 0 0 1 1 1
  line L505 (-19.8336, 12.0346) -> (-19.0547, 12.0346)
  spline S472 degree 2 poles (-19.0547, 12.0346) (-18.9194, 12.0346) (-18.7214, 12.2326) (-18.7214, 12.368) knots 0 0 0 1 2 2 2
  line L506 (-18.7214, 12.368) -> (-18.7214, 12.698)
  spline S473 degree 2 poles (-15.5069, 12.9488) (-15.5069, 12.698) (-15.7577, 12.698) knots 0 0 0 1 1 1
  spline S474 degree 2 poles (-15.7577, 12.698) (-16.0085, 12.698) (-16.0085, 12.9488) knots 0 0 0 1 1 1
  line L507 (-16.0085, 12.9488) -> (-16.0085, 15.0247)
  line L508 (-16.0085, 15.0247) -> (-16.3551, 15.0247)
  line L509 (-16.3551, 15.0247) -> (-17.0812, 12.83)
  spline S475 degree 2 poles (-17.0812, 12.83) (-17.1208, 12.698) (-17.2957, 12.698) knots 0 0 0 1 1 1
  spline S476 degree 2 poles (-17.2957, 12.698) (-17.5531, 12.698) (-17.5531, 12.9389) knots 0 0 0 1 1 1
  spline S477 degree 2 poles (-17.5531, 12.9389) (-17.5531, 12.9851) (-17.5399, 13.028) knots 0 0 0 1 1 1
  line L510 (-17.5399, 13.028) -> (-16.7577, 15.3911)
  spline S478 degree 2 poles (-16.7577, 15.3911) (-16.7181, 15.5231) (-16.5366, 15.5231) knots 0 0 0 1 1 1
  line L511 (-16.5366, 15.5231) -> (-15.7577, 15.5231)
  spline S479 degree 2 poles (-15.7577, 15.5231) (-15.5069, 15.5231) (-15.5069, 15.2723) knots 0 0 0 1 1 1
  line L512 (-15.5069, 15.2723) -> (-15.5069, 12.9488)
  line L513 (-14.3419, 14.3581) -> (-13.6224, 14.3581)
  spline S480 degree 2 poles (-13.6224, 14.3581) (-13.2264, 14.3581) (-12.9821, 14.0478) knots 0 0 0 1 1 1
  spline S481 degree 2 poles (-12.9821, 14.0478) (-12.7874, 13.8597) (-12.7874, 13.5297) knots 0 0 0 1 1 1
  spline S482 degree 2 poles (-12.7874, 13.5297) (-12.7874, 13.193) (-12.9821, 13.0478) knots 0 0 0 1 1 1
  spline S483 degree 2 poles (-12.9821, 13.0478) (-13.2264, 12.698) (-13.6224, 12.698) knots 0 0 0 1 1 1
  line L514 (-13.6224, 12.698) -> (-14.5927, 12.698)
  spline S484 degree 2 poles (-14.5927, 12.698) (-14.8435, 12.698) (-14.8435, 12.9488) knots 0 0 0 1 1 1
  line L515 (-14.8435, 12.9488) -> (-14.8435, 15.2723)
  spline S485 degree 2 poles (-14.8435, 15.2723) (-14.8435, 15.5231) (-14.5927, 15.5231) knots 0 0 0 1 1 1
  spline S486 degree 2 poles (-14.5927, 15.5231) (-14.3419, 15.5231) (-14.3419, 15.2723) knots 0 0 0 1 1 1
  line L516 (-14.3419, 15.2723) -> (-14.3419, 14.3581)
  line L517 (-14.3419, 13.8597) -> (-14.3419, 13.1963)
  line L518 (-14.3419, 13.1963) -> (-13.6224, 13.1963)
  spline S487 degree 2 poles (-13.6224, 13.1963) (-13.464, 13.1963) (-13.3089, 13.3152) knots 0 0 0 1 1 1
  spline S488 degree 2 poles (-13.3089, 13.3152) (-13.2891, 13.3911) (-13.2891, 13.5297) knots 0 0 0 1 1 1
  spline S489 degree 2 poles (-13.2891, 13.5297) (-13.2891, 13.665) (-13.3056, 13.7409) knots 0 0 0 1 1 1
  spline S490 degree 2 poles (-13.3056, 13.7409) (-13.464, 13.8597) (-13.6224, 13.8597) knots 0 0 0 1 1 1
  line L519 (-13.6224, 13.8597) -> (-14.3419, 13.8597)
  line L520 (-10.9656, 15.0247) -> (-11.6257, 15.0247)
  line L521 (-11.6257, 15.0247) -> (-11.6257, 12.9488)
  spline S491 degree 2 poles (-11.6257, 12.9488) (-11.6257, 12.698) (-11.8765, 12.698) knots 0 0 0 1 1 1
  spline S492 degree 2 poles (-11.8765, 12.698) (-12.1274, 12.698) (-12.1274, 12.9488) knots 0 0 0 1 1 1
  line L522 (-12.1274, 12.9488) -> (-12.1274, 15.2723)
  spline S493 degree 2 poles (-12.1274, 15.2723) (-12.1274, 15.5231) (-11.8765, 15.5231) knots 0 0 0 1 1 1
  line L523 (-11.8765, 15.5231) -> (-10.1373, 15.5231)
  spline S494 degree 2 poles (-10.1373, 15.5231) (-9.7907, 15.5231) (-9.3023, 15.0346) (-9.3023, 14.6914) knots 0 0 0 1 2 2 2
  line L524 (-9.3023, 14.6914) -> (-9.3023, 12.9488)
  spline S495 degree 2 poles (-9.3023, 12.9488) (-9.3023, 12.698) (-9.5531, 12.698) knots 0 0 0 1 1 1
  spline S496 degree 2 poles (-9.5531, 12.698) (-9.8039, 12.698) (-9.8039, 12.9488) knots 0 0 0 1 1 1
  line L525 (-9.8039, 12.9488) -> (-9.8039, 14.6947)
  spline S497 degree 2 poles (-9.8039, 14.6947) (-9.8039, 14.8267) (-10.0019, 15.0247) (-10.134, 15.0247) knots 0 0 0 1 2 2 2
  line L526 (-10.134, 15.0247) -> (-10.464, 15.0247)
  line L527 (-10.464, 15.0247) -> (-10.464, 12.9488)
  spline S498 degree 2 poles (-10.464, 12.9488) (-10.464, 12.698) (-10.7148, 12.698) knots 0 0 0 1 1 1
  spline S499 degree 2 poles (-10.7148, 12.698) (-10.9656, 12.698) (-10.9656, 12.9488) knots 0 0 0 1 1 1
  line L528 (-10.9656, 12.9488) -> (-10.9656, 15.0247)
  spline S500 degree 2 poles (2.3379, 9.834) (2.6779, 9.834) (2.9221, 9.5535) knots 0 0 0 1 1 1
  spline S501 degree 2 poles (2.9221, 9.5535) (3.1102, 9.372) (3.1102, 9.0156) knots 0 0 0 1 1 1
  line L529 (3.1102, 9.0156) -> (3.1102, 7.8538)
  spline S502 degree 2 poles (3.1102, 7.8538) (3.1102, 7.5106) (2.6251, 7.0222) (2.2785, 7.0222) knots 0 0 0 1 2 2 2
  line L530 (2.2785, 7.0222) -> (1.8891, 7.0222)
  spline S503 degree 2 poles (1.8891, 7.0222) (1.5492, 7.0222) (1.0607, 7.5073) (1.0607, 7.8538) knots 0 0 0 1 2 2 2
  line L531 (1.0607, 7.8538) -> (1.0607, 10.2565)
  spline S504 degree 2 poles (1.0607, 10.2565) (1.0607, 10.6096) (1.295, 10.8208) knots 0 0 0 1 1 1
  spline S505 degree 2 poles (1.295, 10.8208) (1.5096, 11.009) (1.8165, 11.009) knots 0 0 0 1 1 1
  spline S506 degree 2 poles (1.8165, 11.009) (2.1234, 11.009) (2.2653, 10.8373) knots 0 0 0 1 1 1
  spline S507 degree 2 poles (2.2653, 10.8373) (2.569, 10.6129) (2.569, 10.2598) knots 0 0 0 1 1 1
  spline S508 degree 2 poles (2.569, 10.2598) (2.569, 9.9033) (2.3379, 9.834) knots 0 0 0 1 1 1
  line L532 (2.6086, 7.8505) -> (2.6086, 9.0156)
  spline S509 degree 2 poles (2.6086, 9.0156) (2.6086, 9.1476) (2.4106, 9.3456) (2.2785, 9.3456) knots 0 0 0 1 2 2 2
  line L533 (2.2785, 9.3456) -> (1.8891, 9.3456)
  spline S510 degree 2 poles (1.8891, 9.3456) (1.7571, 9.3456) (1.5624, 9.1509) (1.5624, 9.0156) knots 0 0 0 1 2 2 2
  line L534 (1.5624, 9.0156) -> (1.5624, 7.8505)
  spline S511 degree 2 poles (1.5624, 7.8505) (1.5624, 7.7152) (1.7571, 7.5205) (1.8891, 7.5205) knots 0 0 0 1 2 2 2
  line L535 (1.8891, 7.5205) -> (2.2785, 7.5205)
  spline S512 degree 2 poles (2.2785, 7.5205) (2.4139, 7.5205) (2.6086, 7.7152) (2.6086, 7.8505) knots 0 0 0 1 2 2 2
  spline S513 degree 2 poles (1.5624, 9.7119) (1.6218, 9.7977) (1.8495, 9.9628) knots 0 0 0 1 1 1
  spline S514 degree 2 poles (1.8495, 9.9628) (2.0673, 10.1344) (2.0673, 10.2532) knots 0 0 0 1 1 1
  spline S515 degree 2 poles (2.0673, 10.2532) (2.0673, 10.3753) (1.9782, 10.4545) knots 0 0 0 1 1 1
  spline S516 degree 2 poles (1.9782, 10.4545) (1.9155, 10.504) (1.8132, 10.504) knots 0 0 0 1 1 1
  spline S517 degree 2 poles (1.8132, 10.504) (1.7076, 10.504) (1.6581, 10.4875) knots 0 0 0 1 1 1
  spline S518 degree 2 poles (1.6581, 10.4875) (1.5624, 10.3753) (1.5624, 10.2532) knots 0 0 0 1 1 1
  line L536 (1.5624, 10.2532) -> (1.5624, 9.7119)
  spline S519 degree 2 poles (4.602, 8.2895) (4.5525, 8.2499) (4.2356, 7.8703) knots 0 0 0 1 1 1
  line L537 (4.2356, 7.8703) -> (4.2356, 7.273)
  spline S520 degree 2 poles (4.2356, 7.273) (4.2356, 7.0222) (3.9848, 7.0222) knots 0 0 0 1 1 1
  spline S521 degree 2 poles (3.9848, 7.0222) (3.734, 7.0222) (3.734, 7.273) knots 0 0 0 1 1 1
  line L538 (3.734, 7.273) -> (3.734, 9.5964)
  spline S522 degree 2 poles (3.734, 9.5964) (3.734, 9.8472) (3.9848, 9.8472) knots 0 0 0 1 1 1
  spline S523 degree 2 poles (3.9848, 9.8472) (4.2356, 9.8472) (4.2356, 9.5964) knots 0 0 0 1 1 1
  line L539 (4.2356, 9.5964) -> (4.2356, 8.5106)
  line L540 (4.2356, 8.5106) -> (5.404, 9.7977)
  spline S524 degree 2 poles (5.404, 9.7977) (5.4337, 9.8571) (5.5294, 9.8571) knots 0 0 0 1 1 1
  spline S525 degree 2 poles (5.5294, 9.8571) (5.6317, 9.8571) (5.7802, 9.6921) (5.7802, 9.5931) knots 0 0 0 1 2 2 2
  spline S526 degree 2 poles (5.7802, 9.5931) (5.7802, 9.4875) (5.7043, 9.4116) knots 0 0 0 1 1 1
  line L541 (5.7043, 9.4116) -> (4.9419, 8.6261)
  line L542 (4.9419, 8.6261) -> (5.7241, 7.4347)
  spline S527 degree 2 poles (5.7241, 7.4347) (5.7802, 7.3489) (5.7802, 7.2697) knots 0 0 0 1 1 1
  spline S528 degree 2 poles (5.7802, 7.2697) (5.7802, 7.1641) (5.6218, 7.0156) (5.5261, 7.0156) knots 0 0 0 1 2 2 2
  spline S529 degree 2 poles (5.5261, 7.0156) (5.404, 7.0156) (5.3677, 7.0915) knots 0 0 0 1 1 1
  line L543 (5.3677, 7.0915) -> (4.602, 8.2895)
  spline S530 degree 2 poles (8.5393, 7.273) (8.5393, 7.0222) (8.2884, 7.0222) knots 0 0 0 1 1 1
  spline S531 degree 2 poles (8.2884, 7.0222) (8.0376, 7.0222) (8.0376, 7.273) knots 0 0 0 1 1 1
  line L544 (8.0376, 7.273) -> (8.0376, 9.3489)
  line L545 (8.0376, 9.3489) -> (7.6911, 9.3489)
  line L546 (7.6911, 9.3489) -> (6.965, 7.1542)
  spline S532 degree 2 poles (6.965, 7.1542) (6.9254, 7.0222) (6.7505, 7.0222) knots 0 0 0 1 1 1
  spline S533 degree 2 poles (6.7505, 7.0222) (6.4931, 7.0222) (6.4931, 7.2631) knots 0 0 0 1 1 1
  spline S534 degree 2 poles (6.4931, 7.2631) (6.4931, 7.3093) (6.5063, 7.3522) knots 0 0 0 1 1 1
  line L547 (6.5063, 7.3522) -> (7.2884, 9.7152)
  spline S535 degree 2 poles (7.2884, 9.7152) (7.328, 9.8472) (7.5096, 9.8472) knots 0 0 0 1 1 1
  line L548 (7.5096, 9.8472) -> (8.2884, 9.8472)
  spline S536 degree 2 poles (8.2884, 9.8472) (8.5393, 9.8472) (8.5393, 9.5964) knots 0 0 0 1 1 1
  line L549 (8.5393, 9.5964) -> (8.5393, 7.273)
  line L550 (9.7076, 8.6822) -> (9.9782, 8.6822)
  line L551 (9.9782, 8.6822) -> (9.9782, 9.1311)
  spline S537 degree 2 poles (9.9782, 9.1311) (9.9782, 9.4248) (10.3941, 9.8472) (10.6944, 9.8472) knots 0 0 0 1 2 2 2
  line L552 (10.6944, 9.8472) -> (10.9254, 9.8472)
  spline S538 degree 2 poles (10.9254, 9.8472) (11.2257, 9.8472) (11.6449, 9.4281) (11.6449, 9.1311) knots 0 0 0 1 2 2 2
  line L553 (11.6449, 9.1311) -> (11.6449, 7.7383)
  spline S539 degree 2 poles (11.6449, 7.7383) (11.6449, 7.438) (11.229, 7.0222) (10.9254, 7.0222) knots 0 0 0 1 2 2 2
  line L554 (10.9254, 7.0222) -> (10.6944, 7.0222)
  spline S540 degree 2 poles (10.6944, 7.0222) (10.3941, 7.0222) (9.9782, 7.438) (9.9782, 7.735) knots 0 0 0 1 2 2 2
  line L555 (9.9782, 7.735) -> (9.9782, 8.1839)
  line L556 (9.9782, 8.1839) -> (9.7076, 8.1839)
  line L557 (9.7076, 8.1839) -> (9.7076, 7.273)
  spline S541 degree 2 poles (9.7076, 7.273) (9.7076, 7.0222) (9.4568, 7.0222) knots 0 0 0 1 1 1
  spline S542 degree 2 poles (9.4568, 7.0222) (9.2059, 7.0222) (9.2059, 7.273) knots 0 0 0 1 1 1
  line L558 (9.2059, 7.273) -> (9.2059, 9.5964)
  spline S543 degree 2 poles (9.2059, 9.5964) (9.2059, 9.8472) (9.4568, 9.8472) knots 0 0 0 1 1 1
  spline S544 degree 2 poles (9.4568, 9.8472) (9.7076, 9.8472) (9.7076, 9.5964) knots 0 0 0 1 1 1
  line L559 (9.7076, 9.5964) -> (9.7076, 8.6822)
  line L560 (11.1432, 7.735) -> (11.1432, 9.1344)
  spline S545 degree 2 poles (11.1432, 9.1344) (11.1432, 9.2202) (11.0145, 9.3489) (10.9254, 9.3489) knots 0 0 0 1 2 2 2
  line L561 (10.9254, 9.3489) -> (10.6944, 9.3489)
  spline S546 degree 2 poles (10.6944, 9.3489) (10.6053, 9.3489) (10.4799, 9.2202) (10.4799, 9.1344) knots 0 0 0 1 2 2 2
  line L562 (10.4799, 9.1344) -> (10.4799, 7.735)
  spline S547 degree 2 poles (10.4799, 7.735) (10.4799, 7.6459) (10.6053, 7.5205) (10.6944, 7.5205) knots 0 0 0 1 2 2 2
  line L563 (10.6944, 7.5205) -> (10.9254, 7.5205)
  spline S548 degree 2 poles (10.9254, 7.5205) (11.0145, 7.5205) (11.1432, 7.6459) (11.1432, 7.735) knots 0 0 0 1 2 2 2
  line L564 (13.8594, 8.6822) -> (13.8594, 9.5964)
  spline S549 degree 2 poles (13.8594, 9.5964) (13.8594, 9.8472) (14.1102, 9.8472) knots 0 0 0 1 1 1
  spline S550 degree 2 poles (14.1102, 9.8472) (14.3611, 9.8472) (14.3611, 9.5964) knots 0 0 0 1 1 1
  line L565 (14.3611, 9.5964) -> (14.3611, 7.273)
  spline S551 degree 2 poles (14.3611, 7.273) (14.3611, 7.0222) (14.1102, 7.0222) knots 0 0 0 1 1 1
  spline S552 degree 2 poles (14.1102, 7.0222) (13.8594, 7.0222) (13.8594, 7.273) knots 0 0 0 1 1 1
  line L566 (13.8594, 7.273) -> (13.8594, 8.1839)
  line L567 (13.8594, 8.1839) -> (13.1399, 8.1839)
  spline S553 degree 2 poles (13.1399, 8.1839) (12.7967, 8.1839) (12.3049, 8.669) (12.3049, 9.0156) knots 0 0 0 1 2 2 2
  line L568 (12.3049, 9.0156) -> (12.3049, 9.5964)
  spline S554 degree 2 poles (12.3049, 9.5964) (12.3049, 9.8472) (12.5558, 9.8472) knots 0 0 0 1 1 1